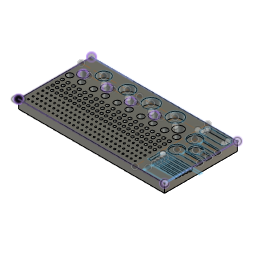
Tools Plate For 3018 Pro v4 (Autodesk Fusion 360 archive; units mm, degrees)
design "Tools Plate For 3018 Pro" references "Commercial Use License & Donation"
Autodesk Fusion 360 part; units mm, degrees
sketch "Wood" plane through (0, 0, 0) normal (0, 0, 1) x (1, 0, 0)
  line L0 (0, 0) -> (300, 0)
  line L1 (300, 0) -> (300, 150)
  line L2 (0, 150) -> (0, 0)
  line L3 (300, 0) -> (300, 150)
  line L4 (300, 150) -> (0, 150)
  dimension "d1" = 300
  dimension "d2" = 150
  constraint horizontal L0
  constraint vertical L1
  constraint vertical L2
  constraint coincident L0.start L2.end
  constraint vertical L3
  constraint coincident L2 L4.end
  constraint perpendicular L2 L4
  measures "d1" distance of L0.start L0.end
  measures "d2" distance of L0.start L2.start
extrude "Extrude1" add sketch "Wood" against normal blind 17.8 makes body 1
sketch "ToolFormat" plane through (0, 0, 0) normal (0, 0, 1) x (1, 0, 0)
  circle A0 centre (0, 0) radius 1.65
  circle A1 centre (0, 0) radius 2.65
  circle A2 centre (0, 0) radius 3.15
  circle A3 centre (0, 0) radius 6.25
  circle A4 centre (0, 0) radius 10
  line L0 (300, 150) -> (300, 0)
  line L1 (0, 0) -> (0, 150)
  point P0 (300, 0)
  dimension "d6" = 3.3
  dimension "d7" = 5.3
  dimension "d8" = 6.3
  dimension "d9" = 12.5
  dimension "d10" = 20
  constraint coincident A0.centre A1.centre
  constraint concentric A0 A1
  constraint concentric A1 A3
  constraint concentric A1 A4
  measures "d6" diameter of A0
  measures "d7" diameter of A1
  measures "d8" diameter of A2
  measures "d9" diameter of A3
  measures "d10" diameter of A4
extrude "Extrude2" add sketch "ToolFormat" against normal blind 14 separate body contours A0 makes body 2
extrude "Extrude3" add sketch "ToolFormat" against normal blind 14 separate body contours A0 | A1 makes body 3
extrude "Extrude4" add sketch "ToolFormat" against normal blind 14 separate body contours A0 | A1 | A2 makes body 4
extrude "Extrude5" add sketch "ToolFormat" against normal blind 15 separate body contours A0 | A1 | A2 | A3 makes body 5
extrude "Extrude6" add sketch "ToolFormat" against normal blind 15 separate body contours A0 | A1 | A2 | A3 | A4 makes body 6
move_body "Move1" bodies 2 to x (1, 0, 0) y (0, 1, 0) z (0, 0, 1) at (10, 10, 0)
pattern_linear "R-Pattern1" count 27 spacing 8.4615 along (1, 0, 0) count 4 spacing 10 along (0, 1, 0) of bodies 2 makes body 7 at (20.1096, 9.919, -9.3333) makes body 8 at (28.5711, 9.919, -9.3333) makes body 9 at (37.0326, 9.919, -9.3333) makes body 10 at (45.4942, 9.919, -9.3333) makes body 11 at (53.9557, 9.919, -9.3333) makes body 12 at (62.4172, 9.919, -9.3333) makes body 13 at (68.5993, 11.5244, -9.3333) makes body 14 at (77.0609, 11.5244, -9.3333) makes body 15 at (85.5224, 11.5244, -9.3333) makes body 16 at (93.984, 11.5244, -9.3333) makes body 17 at (102.4455, 11.5244, -9.3333) makes body 18 at (110.907, 11.5244, -9.3333) makes body 19 at (119.3686, 11.5244, -9.3333) makes body 20 at (128.5425, 8.352, -9.3333) makes body 21 at (137.004, 8.352, -9.3333) makes body 22 at (145.4656, 8.352, -9.3333) makes body 23 at (153.9271, 8.352, -9.3333) makes body 24 at (162.3887, 8.352, -9.3333) makes body 25 at (170.8502, 8.352, -9.3333) makes body 26 at (179.3117, 8.352, -9.3333) makes body 27 at (187.7733, 8.352, -9.3333) makes body 28 at (196.2348, 8.352, -9.3333) makes body 29 at (204.6963, 8.352, -9.3333) makes body 30 at (213.1579, 8.352, -9.3333) makes body 31 at (221.6194, 8.352, -9.3333) makes body 32 at (230.081, 8.352, -9.3333) makes body 33 at (11.648, 19.919, -9.3333) makes body 34 at (20.1096, 19.919, -9.3333) makes body 35 at (28.5711, 19.919, -9.3333) makes body 36 at (37.0326, 19.919, -9.3333) makes body 37 at (45.4942, 19.919, -9.3333) makes body 38 at (53.9557, 19.919, -9.3333) makes body 39 at (62.4172, 19.919, -9.3333) makes body 40 at (68.5993, 21.5244, -9.3333) makes body 41 at (77.0609, 21.5244, -9.3333) makes body 42 at (85.5224, 21.5244, -9.3333) makes body 43 at (93.984, 21.5244, -9.3333) makes body 44 at (102.4455, 21.5244, -9.3333) makes body 45 at (110.907, 21.5244, -9.3333) makes body 46 at (119.3686, 21.5244, -9.3333) makes body 47 at (128.5425, 18.352, -9.3333) makes body 48 at (137.004, 18.352, -9.3333) makes body 49 at (145.4656, 18.352, -9.3333) makes body 50 at (153.9271, 18.352, -9.3333) makes body 51 at (162.3887, 18.352, -9.3333) makes body 52 at (170.8502, 18.352, -9.3333) makes body 53 at (179.3117, 18.352, -9.3333) makes body 54 at (187.7733, 18.352, -9.3333) makes body 55 at (196.2348, 18.352, -9.3333) makes body 56 at (204.6963, 18.352, -9.3333) makes body 57 at (213.1579, 18.352, -9.3333) makes body 58 at (221.6194, 18.352, -9.3333) makes body 59 at (230.081, 18.352, -9.3333) makes body 60 at (11.648, 29.919, -9.3333) makes body 61 at (20.1096, 29.919, -9.3333) makes body 62 at (28.5711, 29.919, -9.3333) makes body 63 at (37.0326, 29.919, -9.3333) makes body 64 at (45.4942, 29.919, -9.3333) makes body 65 at (53.9557, 29.919, -9.3333) makes body 66 at (62.4172, 29.919, -9.3333) makes body 67 at (68.5993, 31.5244, -9.3333) makes body 68 at (77.0609, 31.5244, -9.3333) makes body 69 at (85.5224, 31.5244, -9.3333) makes body 70 at (93.984, 31.5244, -9.3333) makes body 71 at (102.4455, 31.5244, -9.3333) makes body 72 at (110.907, 31.5244, -9.3333) makes body 73 at (119.3686, 31.5244, -9.3333) makes body 74 at (128.5425, 28.352, -9.3333) makes body 75 at (137.004, 28.352, -9.3333) makes body 76 at (145.4656, 28.352, -9.3333) makes body 77 at (153.9271, 28.352, -9.3333) makes body 78 at (162.3887, 28.352, -9.3333) makes body 79 at (170.8502, 28.352, -9.3333) makes body 80 at (179.3117, 28.352, -9.3333) makes body 81 at (187.7733, 28.352, -9.3333) makes body 82 at (196.2348, 28.352, -9.3333) makes body 83 at (204.6963, 28.352, -9.3333) makes body 84 at (213.1579, 28.352, -9.3333) makes body 85 at (221.6194, 28.352, -9.3333) makes body 86 at (230.081, 28.352, -9.3333) makes body 87 at (11.648, 39.919, -9.3333) makes body 88 at (20.1096, 39.919, -9.3333) makes body 89 at (28.5711, 39.919, -9.3333) makes body 90 at (37.0326, 39.919, -9.3333) makes body 91 at (45.4942, 39.919, -9.3333) makes body 92 at (53.9557, 39.919, -9.3333) makes body 93 at (62.4172, 39.919, -9.3333) makes body 94 at (70.8788, 39.919, -9.3333) makes body 95 at (79.3403, 39.919, -9.3333) makes body 96 at (87.8019, 39.919, -9.3333) makes body 97 at (96.2634, 39.919, -9.3333) makes body 98 at (104.7249, 39.919, -9.3333) makes body 99 at (113.1865, 39.919, -9.3333) makes body 100 at (121.648, 39.919, -9.3333) makes body 101 at (128.5425, 38.352, -9.3333) makes body 102 at (137.004, 38.352, -9.3333) makes body 103 at (145.4656, 38.352, -9.3333) makes body 104 at (153.9271, 38.352, -9.3333) makes body 105 at (162.3887, 38.352, -9.3333) makes body 106 at (170.8502, 38.352, -9.3333) makes body 107 at (179.3117, 38.352, -9.3333) makes body 108 at (187.7733, 38.352, -9.3333) makes body 109 at (196.2348, 38.352, -9.3333) makes body 110 at (204.6963, 38.352, -9.3333) makes body 111 at (213.1579, 38.352, -9.3333) makes body 112 at (221.6194, 38.352, -9.3333) makes body 113 at (230.081, 38.352, -9.3333)
move_body "Move2" bodies 3 to x (1, 0, 0) y (0, 1, 0) z (0, 0, 1) at (10, 50, 0)
pattern_linear "R-Pattern2" count 25 spacing 9.1667 along (1, 0, 0) count 2 spacing 10 along (0, 1, 0) of bodies 3 makes body 114 at (21.8135, 49.87, -9.3333) makes body 115 at (30.9801, 49.87, -9.3333) makes body 116 at (40.1468, 49.87, -9.3333) makes body 117 at (49.3135, 49.87, -9.3333) makes body 118 at (58.4801, 49.87, -9.3333) makes body 119 at (67.6468, 49.87, -9.3333) makes body 120 at (76.8135, 49.87, -9.3333) makes body 121 at (85.9801, 49.87, -9.3333) makes body 122 at (95.1468, 49.87, -9.3333) makes body 123 at (104.3135, 49.87, -9.3333) makes body 124 at (113.4801, 49.87, -9.3333) makes body 125 at (122.6468, 49.87, -9.3333) makes body 126 at (129.6837, 47.4009, -9.3333) makes body 127 at (136.6522, 52.0485, -9.3333) makes body 128 at (145.8189, 52.0485, -9.3333) makes body 129 at (155.3043, 52.273, -9.3333) makes body 130 at (164.1522, 52.0485, -9.3333) makes body 131 at (173.3189, 52.0485, -9.3333) makes body 132 at (182.8043, 52.273, -9.3333) makes body 133 at (191.6522, 52.0485, -9.3333) makes body 134 at (200.8189, 52.0485, -9.3333) makes body 135 at (210.3043, 52.273, -9.3333) makes body 136 at (219.1522, 52.0485, -9.3333) makes body 137 at (228.3189, 52.0485, -9.3333) makes body 138 at (12.6468, 59.87, -9.3333) makes body 139 at (21.8135, 59.87, -9.3333) makes body 140 at (30.9801, 59.87, -9.3333) makes body 141 at (40.1468, 59.87, -9.3333) makes body 142 at (49.3135, 59.87, -9.3333) makes body 143 at (58.4801, 59.87, -9.3333) makes body 144 at (67.6468, 59.87, -9.3333) makes body 145 at (76.8135, 59.87, -9.3333) makes body 146 at (85.9801, 59.87, -9.3333) makes body 147 at (95.1468, 59.87, -9.3333) makes body 148 at (104.3135, 59.87, -9.3333) makes body 149 at (113.4801, 59.87, -9.3333) makes body 150 at (122.6468, 59.87, -9.3333) makes body 151 at (129.6837, 57.4009, -9.3333) makes body 152 at (136.6522, 62.0485, -9.3333) makes body 153 at (145.8189, 62.0485, -9.3333) makes body 154 at (155.3043, 62.273, -9.3333) makes body 155 at (164.1522, 62.0485, -9.3333) makes body 156 at (173.3189, 62.0485, -9.3333) makes body 157 at (182.8043, 62.273, -9.3333) makes body 158 at (191.6522, 62.0485, -9.3333) makes body 159 at (200.8189, 62.0485, -9.3333) makes body 160 at (210.3043, 62.273, -9.3333) makes body 161 at (219.1522, 62.0485, -9.3333) makes body 162 at (228.3189, 62.0485, -9.3333)
move_body "Move3" bodies 4 to x (1, 0, 0) y (0, 1, 0) z (0, 0, 1) at (10, 70, 0)
pattern_linear "R-Pattern3" count 20 spacing 11.5789 along (1, 0, 0) count 2 spacing 10 along (0, 1, 0) of bodies 4 makes body 163 at (24.7252, 69.8454, -9.3333) makes body 164 at (36.3041, 69.8454, -9.3333) makes body 165 at (47.883, 69.8454, -9.3333) makes body 166 at (59.462, 69.8454, -9.3333) makes body 167 at (71.0409, 69.8454, -9.3333) makes body 168 at (82.6199, 69.8454, -9.3333) makes body 169 at (94.1988, 69.8454, -9.3333) makes body 170 at (105.7778, 69.8454, -9.3333) makes body 171 at (117.3567, 69.8454, -9.3333) makes body 172 at (128.9357, 69.8454, -9.3333) makes body 173 at (135.749, 67.2982, -9.3333) makes body 174 at (147.3279, 67.2982, -9.3333) makes body 175 at (158.9069, 67.2982, -9.3333) makes body 176 at (170.4858, 67.2982, -9.3333) makes body 177 at (182.0648, 67.2982, -9.3333) makes body 178 at (193.6437, 67.2982, -9.3333) makes body 179 at (205.2227, 67.2982, -9.3333) makes body 180 at (216.8016, 67.2982, -9.3333) makes body 181 at (228.3806, 67.2982, -9.3333) makes body 182 at (13.1462, 79.8454, -9.3333) makes body 183 at (24.7252, 79.8454, -9.3333) makes body 184 at (36.3041, 79.8454, -9.3333) makes body 185 at (47.883, 79.8454, -9.3333) makes body 186 at (59.462, 79.8454, -9.3333) makes body 187 at (71.0409, 79.8454, -9.3333) makes body 188 at (82.6199, 79.8454, -9.3333) makes body 189 at (94.1988, 79.8454, -9.3333) makes body 190 at (105.7778, 79.8454, -9.3333) makes body 191 at (117.3567, 79.8454, -9.3333) makes body 192 at (128.9357, 79.8454, -9.3333) makes body 193 at (135.749, 77.2982, -9.3333) makes body 194 at (147.3279, 77.2982, -9.3333) makes body 195 at (158.9069, 77.2982, -9.3333) makes body 196 at (170.4858, 77.2982, -9.3333) makes body 197 at (182.0648, 77.2982, -9.3333) makes body 198 at (193.6437, 77.2982, -9.3333) makes body 199 at (205.2227, 77.2982, -9.3333) makes body 200 at (216.8016, 77.2982, -9.3333) makes body 201 at (228.3806, 77.2982, -9.3333)
move_body "Move4" bodies 5 to x (1, 0, 0) y (0, 1, 0) z (0, 0, 1) at (10, 95, 0)
pattern_linear "R-Pattern4" count 10 spacing 24.4444 along (1, 0, 0) of bodies 5 makes body 202 at (28.7945, 92.3278, -10) makes body 203 at (53.239, 92.3278, -10) makes body 204 at (84.5526, 88.8701, -10) makes body 205 at (108.9971, 88.8701, -10) makes body 206 at (130.4079, 89.0191, -10) makes body 207 at (154.8524, 89.0191, -10) makes body 208 at (179.2968, 89.0191, -10) makes body 209 at (203.7413, 89.0191, -10) makes body 210 at (228.1857, 89.0191, -10)
move_body "Move5" bodies 6 to x (1, 0, 0) y (0, 1, 0) z (0, 0, 1) at (22, 111, 0)
pattern_linear "R-Pattern5" count 5 spacing 49 along (1, 0, 0) of bodies 6 makes body 211 at (61.1082, 112.4673, -10) makes body 212 at (111.1808, 115.714, -10) makes body 213 at (166.5702, 120.7003, -10) makes body 214 at (215.5702, 120.7003, -10)
sketch "BigHoles" plane through (0, 0, 0) normal (0, 0, 1) x (1, 0, 0)
  line L0 (0, 0) -> (0, 150) construction
  line L1 (0, 128.7407) -> (240, 128.7407) construction
  circle A0 centre (22, 111) radius 10 construction
  circle A1 centre (22, 111) radius 10 construction
  line L2 (31.4551, 114.2559) -> (61.3017, 114.2559) construction
  circle A2 centre (71, 111) radius 10 construction
  circle A3 centre (71, 111) radius 10 construction
  line L3 (80.3943, 114.4274) -> (110.3388, 114.4274) construction
  circle A4 centre (120, 111) radius 10 construction
  circle A5 centre (120, 111) radius 10 construction
  line L4 (129.433, 114.3193) -> (158.4509, 114.3193) construction
  circle A6 centre (169, 111) radius 10 construction
  circle A7 centre (169, 111) radius 10 construction
  line L5 (178.5965, 113.8121) -> (208.2339, 113.8121) construction
  line L6 (46.3784, 114.2559) -> (46.3784, 128.7407) construction
  line L7 (95.3665, 114.4274) -> (95.3665, 128.7407) construction
  line L8 (143.942, 114.3193) -> (143.942, 128.7407) construction
  line L9 (193.4152, 113.8121) -> (193.4152, 128.7407) construction
  circle A8 centre (46.3784, 128.7407) radius 12.5
  circle A9 centre (95.3665, 128.7407) radius 13.5
  circle A10 centre (143.942, 128.7407) radius 15
  circle A11 centre (193.4152, 128.7407) radius 15
  point P0 (120, 128.7407)
  dimension "d58" = 240
  dimension "d59" = 29.0179
  dimension "d60" = 25
  dimension "d61" = 27
  dimension "d62" = 30
  dimension "d63" = 30
  constraint horizontal L1
  constraint coincident L0 L1.start
  constraint midpoint L1 P0
  constraint horizontal L2
  constraint coincident A0 L2.start
  constraint coincident A1 L2.start
  constraint horizontal L3
  constraint coincident A2 L3.start
  constraint coincident A3 L3.start
  constraint horizontal L4
  constraint coincident A4 L4.start
  constraint coincident A5 L4.start
  constraint horizontal L5
  constraint coincident A6 L5.start
  constraint coincident A7 L5.start
  constraint midpoint L2 L6.start
  constraint coincident L1 L6.end
  constraint perpendicular L1 L6
  constraint midpoint L3 L7.start
  constraint coincident L1 L7.end
  constraint perpendicular L1 L7
  constraint midpoint L4 L8.start
  constraint coincident L1 L8.end
  constraint perpendicular L1 L8
  constraint midpoint L5 L9.start
  constraint coincident L1 L9.end
  constraint perpendicular L1 L9
  constraint coincident L6.end A8.centre
  constraint coincident L7.end A9.centre
  constraint coincident L8.end A10.centre
  constraint coincident L9.end A11.centre
  measures "d58" distance of L1.start L1.end
  measures "d59" distance of L4.start L4.end
  measures "d60" diameter of A8
  measures "d61" diameter of A9
  measures "d62" diameter of A10
  measures "d63" diameter of A11
extrude "Extrude7" add sketch "BigHoles" against normal blind 12 separate body makes body 215 at (108.8497, 128.0677, -8) makes body 216 at (158.9233, 127.993, -8) makes body 217 at (58.8629, 128.1176, -8) makes body 218 at (208.3965, 127.993, -8)
copy_body "CopyPasteBodies1" bodies 6 3 5 4 2 makes body 219 makes body 220 makes body 221 makes body 222 makes body 223
combine "Combine1" operation cut target body 1 tool bodies 217 54 12 57 83 131 28 213 136 43 143 45 196 203 14 32 69 135 13 208 176 16 113 118 107 56 178 39 72 200 71 109 42 186 70 218 55 76 198 29 18 47 66 112 44 171 191 82 212 84 67 108 137 61 10 192 96 60 93 151 141 150 222 164 221 127 37 9 65 148 123 125 220 33 115 142 88 153 170 64 110 120 152 111 187 146 24 7 130 160 62 194 204 19 35 206 122 145 216 181 175 209 215 98 155 197 154 166 8 95 173 169 128 190 174 11 185 162 177 211 183 223 36 129 167 34 182 219 195 63 99 172 38 116 97 91 87 168 184 126 117 94 89 139 163 165 207 114 92 140 90 138 202 22 59 41 103 46 68 158 20 53 134 81 104 27 86 51 199 101 133 17 15 78 25 179 40 106 31 75 157 180 105 21 26 50 30 77 23 100 85 102 161 58 48 159 132 52 214 80 121 79 49 188 147 210 74 144 201 119 73 205 193 124 149 189 156
sketch "KeyHallenAnd Others" plane through (0, 0, 0) normal (0, 0, 1) x (1, 0, 0)
  line L0 (246.9158, 56.8692) -> (319.9158, 56.8692)
  line L1 (319.9158, 56.8692) -> (319.9158, 51.8692)
  line L2 (319.9158, 51.8692) -> (246.9158, 51.8692)
  line L3 (244.9158, 51.8692) -> (244.9158, 56.8692) construction
  line L4 (244.9158, 51.8692) -> (239.9158, 51.8692) construction
  line L5 (239.9158, 49.8692) -> (239.9158, 26.8692)
  line L6 (239.9158, 26.8692) -> (244.9158, 26.8692)
  line L7 (244.9158, 26.8692) -> (244.9158, 49.8692)
  arc A0 (246.9158, 56.8692) -> (239.9158, 49.8692) centre (246.9158, 49.8692) ccw
  arc A1 (246.9158, 51.8692) -> (244.9158, 49.8692) centre (246.9158, 49.8692) ccw
  line L8 (300, 0) -> (0, 0)
  line L9 (0, 150) -> (300, 150)
  line L10 (239.0732, 0) -> (239.0732, 150) construction
  line L11 (300, 51.8692) -> (300, 48.8692)
  line L12 (300, 48.8692) -> (255, 48.8692)
  line L13 (255, 48.8692) -> (255, 43.8692)
  line L14 (255, 43.8692) -> (300, 43.8692)
  line L15 (300, 43.8692) -> (300, 48.8692)
  line L16 (300, 43.8692) -> (300, 40.8692)
  line L17 (300, 40.8692) -> (255, 40.8692)
  line L18 (255, 40.8692) -> (255, 36.3692)
  line L19 (255, 36.3692) -> (300, 36.3692)
  line L20 (300, 36.3692) -> (300, 40.8692)
  line L21 (300, 36.3692) -> (300, 33.3692)
  line L22 (300, 33.3692) -> (300, 29.3692)
  line L23 (300, 29.3692) -> (300, 26.3692)
  line L24 (300, 26.3692) -> (300, 22.8692)
  line L25 (300, 22.8692) -> (300, 19.8692)
  line L26 (300, 19.8692) -> (300, 16.8692)
  line L27 (300, 150) -> (300, 0)
  line L28 (300, 16.8692) -> (300, 13.8692)
  line L29 (300, 13.8692) -> (300, 11.3692)
  line L30 (300, 11.3692) -> (300, 9.3692)
  line L31 (300, 9.3692) -> (300, 7.8692)
  line L32 (300, 7.8692) -> (300, 5.8692)
  line L33 (300, 5.8692) -> (300, 4.8692)
  line L34 (300, 4.8692) -> (300, 2.8692)
  line L35 (300, 2.8692) -> (300, 1.8692)
  line L36 (300, 33.3692) -> (255, 33.3692)
  line L37 (255, 33.3692) -> (255, 29.3692)
  line L38 (255, 29.3692) -> (300, 29.3692)
  line L39 (300, 29.3692) -> (300, 33.3692)
  line L40 (300, 26.3692) -> (255, 26.3692)
  line L41 (255, 26.3692) -> (255, 22.8692)
  line L42 (255, 22.8692) -> (300, 22.8692)
  line L43 (300, 22.8692) -> (300, 26.3692)
  line L44 (300, 19.8692) -> (255, 19.8692)
  line L45 (255, 19.8692) -> (255, 3.3692)
  line L46 (255, 3.3692) -> (300, 3.3692)
  line L47 (300, 3.3692) -> (300, 19.8692)
  circle A2 centre (255, 46.3692) radius 2.5
  circle A3 centre (255, 38.6192) radius 2.25
  circle A4 centre (255, 31.3692) radius 2
  circle A5 centre (255, 24.6192) radius 1.75
  circle A6 centre (252.3511, 73.1987) radius 13
  circle A7 centre (252.3511, 110.1987) radius 13
  line L48 (252.3511, 110.1987) -> (252.3511, 73.1987) construction
  circle A8 centre (273.0725, 91.6779) radius 11
  line L49 (273.0725, 91.6779) -> (300, 91.6779) construction
  line L50 (252.3511, 110.1987) -> (300, 110.1987) construction
  line L51 (252.3511, 73.1987) -> (300, 73.1987) construction
  line L52 (300, 110.1987) -> (300, 116.1987) construction
  line L53 (300, 110.1987) -> (300, 104.1987) construction
  line L54 (300, 91.6779) -> (300, 97.6779) construction
  line L55 (300, 91.6779) -> (300, 85.6779) construction
  line L56 (300, 73.1987) -> (300, 79.1987) construction
  line L57 (300, 73.1987) -> (300, 67.1987) construction
  line L58 (300, 116.1987) -> (263.8836, 116.1987)
  line L59 (300, 104.1987) -> (263.8836, 104.1987)
  line L60 (300, 97.6779) -> (282.292, 97.6779)
  line L61 (300, 85.6779) -> (282.292, 85.6779)
  line L62 (300, 79.1987) -> (263.8836, 79.1987)
  line L63 (300, 67.1987) -> (263.8836, 67.1987)
  line L64 (247.8375, 126.3431) -> (290.9819, 126.3431)
  line L65 (295.9819, 131.3431) -> (295.9819, 140.552)
  line L66 (290.9819, 145.552) -> (247.8375, 145.552)
  line L67 (242.8375, 140.552) -> (242.8375, 131.3431)
  arc A9 (247.8375, 145.552) -> (242.8375, 140.552) centre (247.8375, 140.552) ccw
  arc A10 (242.8375, 131.3431) -> (247.8375, 126.3431) centre (247.8375, 131.3431) ccw
  arc A11 (290.9819, 126.3431) -> (295.9819, 131.3431) centre (290.9819, 131.3431) ccw
  arc A12 (295.9819, 140.552) -> (290.9819, 145.552) centre (290.9819, 140.552) ccw
  line L68 (256.55, 19.8692) -> (253.45, 19.8692)
  line L69 (253.45, 19.8692) -> (253.45, 3.3692)
  line L70 (253.45, 3.3692) -> (256.55, 3.3692)
  line L71 (256.55, 3.3692) -> (256.55, 19.8692)
  line L72 (256.55, 19.8692) -> (253.45, 3.3692) construction
  line L73 (253.45, 19.8692) -> (256.55, 3.3692) construction
  point P0 (286.5362, 91.6779)
  point P1 (255, 11.6192)
  dimension "d66" = 75
  dimension "d67" = 5
  dimension "d70" = 5
  dimension "d71" = 25
  dimension "d73" = 7
  dimension "d74" = 2
  dimension "d75" = 3
  dimension "d76" = 5
  dimension "d77" = 3
  dimension "d78" = 4.5
  dimension "d79" = 3
  dimension "d80" = 4
  dimension "d81" = 3
  dimension "d82" = 3.5
  dimension "d83" = 3
  dimension "d84" = 3
  dimension "d85" = 3
  dimension "d86" = 2.5
  dimension "d87" = 2
  dimension "d88" = 1.5
  dimension "d89" = 2
  dimension "d90" = 1
  dimension "d91" = 2
  dimension "d92" = 1
  dimension "d93" = 45
  dimension "d94" = 45
  dimension "d95" = 3.5
  dimension "d96" = 45
  dimension "d101" = 45
  dimension "d102" = 45
  dimension "d104" = 3.5
  dimension "d105" = 4
  dimension "d106" = 4.5
  dimension "d107" = 5
  dimension "d108" = 26
  dimension "d109" = 26
  dimension "d110" = 22
  dimension "d112" = 6
  dimension "d113" = 6
  dimension "d114" = 6
  dimension "d115" = 6
  dimension "d116" = 6
  dimension "d117" = 6
  dimension "d118" = 5
  dimension "d139" = 3.1
  constraint horizontal L0
  constraint vertical L1
  constraint horizontal L2
  constraint vertical L3
  constraint horizontal L4
  constraint vertical L5
  constraint horizontal L6
  constraint vertical L7
  constraint coincident L3.start L7
  constraint coincident L3.start L2
  constraint coincident L3.end L0
  constraint coincident L4.end L5
  constraint tangent L0 A0
  constraint tangent L5 A0
  constraint tangent L7 A1
  constraint tangent L2 A1
  constraint coincident L8 L10.start
  constraint coincident L9 L10.end
  constraint perpendicular L2 L10
  constraint coincident L2 L11.start
  constraint perpendicular L2 L11
  constraint horizontal L12
  constraint vertical L13
  constraint horizontal L14
  constraint vertical L15
  constraint perpendicular L14 L16
  constraint horizontal L17
  constraint vertical L18
  constraint horizontal L19
  constraint vertical L20
  constraint perpendicular L19 L21
  constraint parallel L21 L22
  constraint parallel L22 L23
  constraint parallel L23 L24
  constraint parallel L24 L25
  constraint parallel L25 L26
  constraint parallel L27 L28
  constraint parallel L27 L29
  constraint parallel L27 L30
  constraint parallel L27 L31
  constraint parallel L27 L32
  constraint parallel L27 L33
  constraint parallel L27 L34
  constraint parallel L27 L35
  constraint horizontal L36
  constraint vertical L37
  constraint horizontal L38
  constraint vertical L39
  constraint horizontal L40
  constraint vertical L41
  constraint horizontal L42
  constraint vertical L43
  constraint horizontal L44
  constraint vertical L45
  constraint horizontal L46
  constraint vertical L47
  constraint midpoint L13 A2.centre
  constraint midpoint L18 A3.centre
  constraint midpoint L37 A4.centre
  constraint midpoint L41 A5.centre
  constraint coincident A7.centre L48.start
  constraint coincident A6.centre L48.end
  constraint vertical L48
  constraint coincident A8.centre L49.start
  constraint coincident L27 L49.end
  constraint perpendicular L27 L49
  constraint coincident L27 L50.end
  constraint perpendicular L27 L50
  constraint coincident L27 L51.end
  constraint perpendicular L27 L51
  constraint midpoint L49 P0
  constraint perpendicular L50 L52
  constraint perpendicular L50 L53
  constraint perpendicular L49 L54
  constraint perpendicular L49 L55
  constraint perpendicular L51 L56
  constraint perpendicular L51 L57
  constraint coincident A7 L58.end
  constraint perpendicular L52 L58
  constraint coincident A7 L59.end
  constraint perpendicular L27 L59
  constraint coincident A8 L60.end
  constraint perpendicular L27 L60
  constraint coincident A8 L61.end
  constraint perpendicular L55 L61
  constraint coincident A6 L62.end
  constraint perpendicular L27 L62
  constraint coincident A6 L63.end
  constraint perpendicular L27 L63
  constraint horizontal L64
  constraint vertical L65
  constraint horizontal L66
  constraint vertical L67
  constraint tangent L66 A9
  constraint tangent L67 A9
  constraint tangent L67 A10
  constraint tangent L64 A10
  constraint equal A9 A10
  constraint tangent L64 A11
  constraint tangent L65 A11
  constraint equal A9 A11
  constraint tangent L65 A12
  constraint tangent L66 A12
  constraint equal A9 A12
  constraint horizontal L68
  constraint perpendicular L68 L69
  constraint parallel L68 L70
  constraint parallel L69 L71
  constraint coincident L72 P1
  constraint coincident L73 P1
  constraint midpoint L45 P1
  measures "d66" distance of L3.end L0.end
  measures "d67" distance of L3.end L3.start
  measures "d70" distance of L3.start L4.end
  measures "d71" distance of L3.start L6.end
  measures "d73" radius of A0
  measures "d74" radius of A1
  measures "d75" distance of L11.start L11.end
  measures "d76" distance of L11.end L14.end
  measures "d77" distance of L14.end L16.end
  measures "d78" distance of L16.end L19.end
  measures "d79" distance of L19.end L21.end
  measures "d80" distance of L21.end L22.end
  measures "d81" distance of L22.end L23.end
  measures "d82" distance of L23.end L24.end
  measures "d83" distance of L24.end L25.end
  measures "d84" distance of L25.end L26.end
  measures "d85" distance of L26.end L28.end
  measures "d86" distance of L28.end L29.end
  measures "d87" distance of L29.end L30.end
  measures "d88" distance of L30.end L31.end
  measures "d89" distance of L31.end L32.end
  measures "d90" distance of L32.end L33.end
  measures "d91" distance of L33.end L34.end
  measures "d92" distance of L34.end L35.end
  measures "d93" distance of L21.end L36.end
  measures "d94" distance of L23.end L40.end
  measures "d95" distance of L23.end L24.end
  measures "d96" distance of L25.end L44.end
  measures "d101" distance of L16.end L17.end
  measures "d102" distance of L11.end L12.end
  measures "d104" diameter of A5
  measures "d105" diameter of A4
  measures "d106" diameter of A3
  measures "d107" diameter of A2
  measures "d108" diameter of A6
  measures "d109" diameter of A7
  measures "d110" diameter of A8
  measures "d112" distance of L50.end L52.end
  measures "d113" distance of L50.end L53.end
  measures "d114" distance of L49.end L54.end
  measures "d115" distance of L49.end L55.end
  measures "d116" distance of L51.end L56.end
  measures "d117" distance of L51.end L57.end
  measures "d118" radius of A9
  measures "d139" distance of L69.end L70.end
extrude "Extrude8" cut sketch "KeyHallenAnd Others" against normal blind 8 contours L64 L65 L66 L67 A9 A10 A11 A12 bodies 1
extrude "Extrude9" cut sketch "KeyHallenAnd Others" against normal blind 3 contours L27 A7 L58 L59 | A7 | L27 A8 L60 L61 | A8 | L27 A6 L62 L63 | A6 bodies 1
extrude "Extrude10" cut sketch "KeyHallenAnd Others" against normal blind 6 contours L0 L2 L5 L6 L7 A0 A1 L27 bodies 1
extrude "Extrude11" cut sketch "KeyHallenAnd Others" against normal blind 5 contours L12 L14 L15 L27 A2 | L13 A2 | L13 A2 bodies 1
extrude "Extrude12" cut sketch "KeyHallenAnd Others" against normal blind 4.5 contours L17 L19 L20 L27 A3 | L18 A3 | L18 A3 bodies 1
extrude "Extrude13" cut sketch "KeyHallenAnd Others" against normal blind 4 contours L22 L27 L36 L38 L39 A4 | L37 A4 | L37 A4 bodies 1
extrude "Extrude14" cut sketch "KeyHallenAnd Others" against normal blind 3.5 contours L24 L27 L40 L42 L43 A5 | L41 A5 | L41 A5 bodies 1
extrude "Extrude18" [rolled back] along distance -3 taper angle 0
extrude "Extrude19" [rolled back] along distance -16 taper angle 0
hidden bodies 2 3 4 5 6
named bodies: "WoodBlock", "3mm", "5mm", "6mm", "12mm", "20mm", "3mm (1)", "3mm (2)", "3mm (3)", "3mm (4)", "3mm (5)", "3mm (6)", "3mm (7)", "3mm (8)", "3mm (9)", "3mm (10)", "3mm (11)", "3mm (12)", "3mm (13)", "3mm (14)", "3mm (15)", "3mm (16)", "3mm (17)", "3mm (18)", "3mm (19)", "3mm (20)", "3mm (21)", "3mm (22)", "3mm (23)", "3mm (24)", "3mm (25)", "3mm (26)", "3mm (27)", "3mm (28)", "3mm (29)", "3mm (30)", "3mm (31)", "3mm (32)", "3mm (33)", "3mm (34)", "3mm (35)", "3mm (36)", "3mm (37)", "3mm (38)", "3mm (39)", "3mm (40)", "3mm (41)", "3mm (42)", "3mm (43)", "3mm (44)", "3mm (45)", "3mm (46)", "3mm (47)", "3mm (48)", "3mm (49)", "3mm (50)", "3mm (51)", "3mm (52)", "3mm (53)", "3mm (54)", "3mm (55)", "3mm (56)", "3mm (57)", "3mm (58)", "3mm (59)", "3mm (60)", "3mm (61)", "3mm (62)", "3mm (63)", "3mm (64)", "3mm (65)", "3mm (66)", "3mm (67)", "3mm (68)", "3mm (69)", "3mm (70)", "3mm (71)", "3mm (72)", "3mm (73)", "3mm (74)", "3mm (75)", "3mm (76)", "3mm (77)", "3mm (78)", "3mm (79)", "3mm (80)", "3mm (81)", "3mm (82)", "3mm (83)", "3mm (84)", "3mm (85)", "3mm (86)", "3mm (87)", "3mm (88)", "3mm (89)", "3mm (90)", "3mm (91)", "3mm (92)", "3mm (93)", "3mm (94)", "3mm (95)", "3mm (96)", "3mm (97)", "3mm (98)", "3mm (99)", "3mm (100)", "3mm (101)", "3mm (102)", "3mm (103)", "3mm (104)", "3mm (105)", "3mm (106)", "3mm (107)", "5mm (1)", "5mm (2)", "5mm (3)", "5mm (4)", "5mm (5)", "5mm (6)", "5mm (7)", "5mm (8)", "5mm (9)", "5mm (10)", "5mm (11)", "5mm (12)", "5mm (13)", "5mm (14)", "5mm (15)", "5mm (16)", "5mm (17)", "5mm (18)", "5mm (19)", "5mm (20)", "5mm (21)", "5mm (22)", "5mm (23)", "5mm (24)", "5mm (25)", "5mm (26)", "5mm (27)", "5mm (28)", "5mm (29)", "5mm (30)", "5mm (31)", "5mm (32)", "5mm (33)", "5mm (34)", "5mm (35)", "5mm (36)", "5mm (37)", "5mm (38)", "5mm (39)", "5mm (40)", "5mm (41)", "5mm (42)", "5mm (43)", "5mm (44)", "5mm (45)", "5mm (46)", "5mm (47)", "5mm (48)", "5mm (49)", "6mm (1)", "6mm (2)", "6mm (3)", "6mm (4)", "6mm (5)", "6mm (6)", "6mm (7)", "6mm (8)", "6mm (9)", "6mm (10)", "6mm (11)", "6mm (12)", "6mm (13)", "6mm (14)", "6mm (15)", "6mm (16)", "6mm (17)", "6mm (18)", "6mm (19)", "6mm (20)", "6mm (21)", "6mm (22)", "6mm (23)", "6mm (24)", "6mm (25)", "6mm (26)", "6mm (27)", "6mm (28)", "6mm (29)", "6mm (30)", "6mm (31)", "6mm (32)", "6mm (33)", "6mm (34)", "6mm (35)", "6mm (36)", "6mm (37)", "6mm (38)", "6mm (39)", "12mm (1)", "12mm (2)", "12mm (3)", "12mm (4)", "12mm (5)", "12mm (6)", "12mm (7)", "12mm (8)", "12mm (9)", "20mm (1)", "20mm (2)", "20mm (3)", "20mm (4)", "20mm (5)", "5mm (50)", "12mm (10)", "6mm (40)", "3mm (108)"
